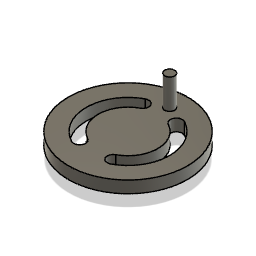
Quick Return Mechanism_ (Autodesk Fusion 360 design; units mm, degrees)
Autodesk Fusion 360 part; units mm, degrees
sketch "Sketch1" plane through (0, 0, 0) normal (0, 1, 0) x (1, 0, 0) in component "Fixed"
  arc A0 (32.0259, -54.4608) -> (60, 0) centre (-7, 0) ccw
  arc A1 (32.0259, -54.4608) -> (3, -110.75) centre (72.5197, -110.97) ccw
  line L0 (3, -110.75) -> (0, -110.75)
  line L1 (0, -110.75) -> (0, 0) construction
  circle A2 centre (30, -20) radius 15
  line L2 (0, -50.75) -> (25, -50.75)
  arc A3 (25, -50.75) -> (25, -40.75) centre (25, -45.75) ccw
  line L3 (25, -40.75) -> (15, -40.75)
  arc A4 (10, -35.75) -> (15, -40.75) centre (15, -35.75) ccw
  line L4 (10, -35.75) -> (10, -15.75)
  arc A5 (10, -15.75) -> (0, -5.75) centre (0, -15.75) ccw
  line L5 (30, -45.75) -> (30, -20) construction
  line L6 (60, 0) -> (0, 0)
  line L7 (0, 0) -> (0, 11.5) construction
  line L8 (0, 11.5) -> (60, 11.5)
  line L9 (60, 11.5) -> (60, 0)
  line L10 (60, 9) -> (0, 9)
  circle A6 centre (0, -65.75) radius 6
  circle A7 centre (0, -100.75) radius 2.05
  line L11 (-2.5, -78.25) -> (-2.5, -93.25)
  arc A8 (-2.5, -93.25) -> (2.5, -93.25) centre (0, -93.25) ccw
  line L12 (2.5, -93.25) -> (2.5, -78.25)
  arc A9 (2.5, -78.25) -> (-2.5, -78.25) centre (0, -78.25) ccw
  line L13 (0, -78.25) -> (0, -93.25) construction
  line L14 (-3, -110.75) -> (0, -110.75)
  arc A10 (-3, -110.75) -> (-32.0259, -54.4608) centre (-72.5197, -110.97) ccw
  arc A11 (-60, 0) -> (-32.0259, -54.4608) centre (7, 0) ccw
  arc A12 (-25, -40.75) -> (-25, -50.75) centre (-25, -45.75) ccw
  line L15 (-25, -40.75) -> (-15, -40.75)
  arc A13 (-15, -40.75) -> (-10, -35.75) centre (-15, -35.75) ccw
  line L16 (-10, -35.75) -> (-10, -15.75)
  arc A14 (0, -5.75) -> (-10, -15.75) centre (0, -15.75) ccw
  line L17 (0, -50.75) -> (-25, -50.75)
  circle A15 centre (-30, -20) radius 15
  line L18 (-60, 0) -> (0, 0)
  line L19 (-60, 9) -> (0, 9)
  line L20 (0, 11.5) -> (-60, 11.5)
  line L21 (-60, 11.5) -> (-60, 0)
  point P0 (0, -85.75)
  dimension "d1" = 7
  dimension "d2" = 67
  dimension "d3" = 69.52
  dimension "d4" = 110.75
  dimension "d5" = 3
  dimension "d6" = 30
  dimension "d7" = 20
  dimension "d8" = 5
  dimension "d9" = 10
  dimension "d10" = 5
  dimension "d11" = 10
  dimension "d12" = 25
  dimension "d13" = 15.75
  dimension "d14" = 90.75
  dimension "d15" = 11.5
  dimension "d16" = 9
  dimension "d17" = 12
  dimension "d18" = 4.1
  dimension "d19" = 2.5
  dimension "d20" = 10
  dimension "d21" = 15
  dimension "d22" = 45
  dimension "d23" = 25
  constraint tangent A0 A1
  constraint horizontal L1.end A0.centre
  constraint horizontal L0
  constraint coincident L1.end L6.end
  constraint vertical L1
  constraint horizontal L1.end A0.end
  constraint coincident L1 L2.start
  constraint perpendicular L1 L2
  constraint tangent L2 A3
  constraint tangent A3 L3
  constraint parallel L2 L3
  constraint tangent L3 A4
  constraint tangent A4 L4
  constraint coincident L1 A5.end
  constraint tangent L4 A5
  constraint vertical L4
  constraint midpoint A3 L5.start
  constraint coincident A2.centre L5.end
  constraint vertical L5
  constraint horizontal L6
  constraint vertical L7
  constraint horizontal L8
  constraint vertical L9
  constraint coincident L1.end L7
  constraint coincident L9 L10.start
  constraint coincident L7 L10.end
  constraint perpendicular L7 L10
  constraint coincident L1 A6.centre
  constraint coincident L1 A7.centre
  constraint tangent L11 A8
  constraint tangent A8 L12
  constraint parallel L11 L12
  constraint tangent L12 A9
  constraint tangent L11 A9
  constraint coincident L1 A8.centre
  constraint parallel L1 L13
  constraint coincident L1 P0
  constraint midpoint L13 P0
  constraint symmetric A0.start L7 A10.end
  constraint symmetric A0.end L7 A11.start
  constraint symmetric A0 L7 A11
  constraint symmetric A1.end L7 L14.start
  constraint symmetric A1 L7 A10
  constraint symmetric L0.end L7 L1.start
  constraint symmetric A2 L7 A15
  constraint symmetric L2.start L7 L17.start
  constraint symmetric L2.end L7 A12.end
  constraint symmetric A3.end L7 A12.start
  constraint symmetric A3 L7 A12
  constraint symmetric L3.end L7 L15.end
  constraint symmetric A4.start L7 A13.end
  constraint symmetric A4 L7 A13
  constraint symmetric L4.end L7 L16.end
  constraint symmetric A5.end L7 A14.start
  constraint symmetric A5 L7 A14
  constraint symmetric L1.end L7 L6.end
  constraint symmetric L8.start L7 L20.start
  constraint symmetric L8.end L7 L20.end
  constraint symmetric L7 L10.start L19.start
  constraint symmetric L7 L10.end L19.end
  measures "d1" distance of L1.end A0.centre
  measures "d2" radius of A0
  measures "d3" radius of A1
  measures "d4" vertical distance of L1.end A1.end
  measures "d5" distance of A1.end L0.end
  measures "d6" diameter of A2
  measures "d7" distance of A4.start L4.end
  measures "d8" radius of A3
  measures "d9" distance of A3.end L3.end
  measures "d10" radius of A4
  measures "d11" radius of A5
  measures "d12" distance of L2.start L2.end
  measures "d13" distance of L1.end A5.centre
  measures "d14" vertical distance of A1.end A2.centre
  measures "d15" distance of A0.end L8.end
  measures "d16" distance of A0.end L10
  measures "d17" diameter of A6
  measures "d18" diameter of A7
  measures "d19" radius of A9
  measures "d20" vertical distance of A1.end A7.centre
  measures "d21" distance of A8.end L12.end
  measures "d22" vertical distance of A1.end A6.centre
  measures "d23" vertical distance of A1.end P0
extrude "Extrude1" add sketch "Sketch1" along normal blind 5 contours A0 A1 L0 L6 L14 A10 A11 L18 | L6 L9 L10 L18 L19 L21 | L8 L9 L10 L19 L20 L21 | A7 makes body 1 in component "Fixed"
extrude "Extrude2" cut sketch "Sketch1" against normal blind 2.5 from surface at 5 contours L6 L9 L10 L18 L19 L21 bodies 1 in component "Fixed"
extrude "Extrude3" add sketch "Sketch1" along normal blind 25 contours A7 bodies 1 in component "Fixed"
sketch "Sketch1 (2)" plane through (0, 0, 0) normal (0, 1, 0) x (1, 0, 0) in component "Crank"
  circle A0 centre (0, -65.75) radius 6
  circle A1 centre (0, -65.75) radius 5.65
  dimension "d31" = 11.3
  constraint concentric A0 A1
  measures "d31" diameter of A1
extrude "Extrude1'" add sketch "Sketch1 (2)" along normal blind 5 separate body contours A1 makes body 2 in component "Crank"
sketch "Sketch2" plane through (0, 5, 0) normal (0, 1, 0) x (-1, 0, 0) in component "Crank"
  circle A0 centre (0, 65.75) radius 5.65
  circle A1 centre (0, 65.75) radius 25
  arc A2 (-8.2158, 81.2016) -> (-8.2158, 50.2984) centre (0, 65.75) ccw
  arc A3 (-5.8684, 76.7868) -> (-8.2158, 81.2016) centre (-7.0421, 78.9942) ccw
  arc A4 (-5.8684, 76.7868) -> (-5.8684, 54.7132) centre (0, 65.75) ccw
  arc A5 (-8.2158, 50.2984) -> (-5.8684, 54.7132) centre (-7.0421, 52.5058) ccw
  arc A6 (-7.0421, 78.9942) -> (-7.0421, 52.5058) centre (0, 65.75) ccw construction
  line L0 (-7.0421, 52.5058) -> (0, 65.75) construction
  line L1 (0, 65.75) -> (-7.0421, 78.9942) construction
  line L2 (0, 65.75) -> (0, 40.75) construction
  arc A7 (5.8684, 54.7132) -> (8.2158, 50.2984) centre (7.0421, 52.5058) ccw
  arc A8 (8.2158, 50.2984) -> (8.2158, 81.2016) centre (0, 65.75) ccw
  arc A9 (8.2158, 81.2016) -> (5.8684, 76.7868) centre (7.0421, 78.9942) ccw
  arc A10 (5.8684, 54.7132) -> (5.8684, 76.7868) centre (0, 65.75) ccw
  line L3 (7.0421, 52.5058) -> (0, 65.75) construction
  circle A11 centre (0, 48.25) radius 2.1
  dimension "d34" = 50
  dimension "d35" = 124
  dimension "d36" = 17.5
  dimension "d37" = 12.5
  dimension "d38" = 56
  dimension "d39" = 4.2
  dimension "d40" = 17.5
  constraint concentric A0 A1
  constraint tangent A2 A3
  constraint tangent A3 A4
  constraint tangent A4 A5
  constraint tangent A2 A5
  constraint coincident A0.centre A1.centre
  constraint coincident A5.centre A6.end
  constraint coincident A3.centre A6.start
  constraint coincident A1 L2.end
  constraint vertical L2
  constraint symmetric A2.end L2 A7.end
  constraint symmetric A2.start L2 A8.end
  constraint symmetric A3.start L2 A9.end
  constraint symmetric A4.end L2 A7.start
  constraint symmetric A2 L2 A8
  constraint symmetric A3 L2 A9
  constraint symmetric A4 L2 A10
  constraint symmetric A5 L2 A7
  constraint symmetric A5.centre L2 A7.centre
  constraint symmetric A0.centre L2 A1.centre
  constraint coincident L2 A11.centre
  measures "d34" diameter of A1
  measures "d35" angle of L0 L1
  measures "d36" radius of A2
  measures "d37" radius of A4
  measures "d38" angle of L0 L3
  measures "d39" diameter of A11
  measures "d40" distance of A0.centre A11.centre
extrude "Extrude2'" add sketch "Sketch2" along normal blind 5 separate body contours A0 | A1 | A11 makes body 3 in component "Crank"
extrude "Extrude3'" add sketch "Sketch2" along normal blind 17.5 contours A11 bodies 3 in component "Crank"
sketch "Sketch1 (3)" plane through (0, 10, 0) normal (0, 1, 0) x (-1, 0, 0) in component "FrontLever"
  circle A0 centre (0, 48.25) radius 2.1
  arc A1 (-5.8684, 76.7868) -> (-8.2158, 81.2016) centre (-7.0421, 78.9942) ccw
  arc A2 (-5.8684, 76.7868) -> (-5.8684, 54.7132) centre (0, 65.75) ccw
  arc A3 (-8.2158, 50.2984) -> (-5.8684, 54.7132) centre (-7.0421, 52.5058) ccw
  arc A4 (-8.2158, 81.2016) -> (-8.2158, 50.2984) centre (0, 65.75) ccw
  arc A5 (8.2158, 50.2984) -> (8.2158, 81.2016) centre (0, 65.75) ccw
  arc A6 (5.8684, 54.7132) -> (8.2158, 50.2984) centre (7.0421, 52.5058) ccw
  arc A7 (5.8684, 54.7132) -> (5.8684, 76.7868) centre (0, 65.75) ccw
  arc A8 (8.2158, 81.2016) -> (5.8684, 76.7868) centre (7.0421, 78.9942) ccw
  circle A9 centre (0, 65.75) radius 25
  circle A10 centre (0, 100.75) radius 2.05
  circle A11 centre (0, 100.75) radius 2.5
  line L0 (6.5, 20.75) -> (-6.5, 20.75)
  line L1 (-6.5, 20.75) -> (-6.5, 100.75)
  line L2 (6.5, 100.75) -> (6.5, 20.75)
  arc A12 (6.5, 100.75) -> (-6.5, 100.75) centre (0, 100.75) ccw
  arc A13 (-2.5, 94.75) -> (2.5, 94.75) centre (0, 100.75) ccw
  line L3 (2.5, 94.75) -> (-2.5, 94.75)
  line L4 (-2.5, 94.75) -> (-2.5, 33.25)
  line L5 (-2.5, 33.25) -> (2.5, 33.25)
  line L6 (2.5, 33.25) -> (2.5, 94.75)
  circle A14 centre (0, 26.25) radius 2.25
  dimension "d45" = 5
  dimension "d47" = 13
  dimension "d48" = 6.5
  dimension "d49" = 5
  dimension "d50" = 12.5
  dimension "d51" = 61.5
  dimension "d52" = 4.5
  dimension "d53" = 5.5
  constraint concentric A10 A11
  constraint horizontal L0
  constraint vertical L1
  constraint vertical L2
  constraint tangent L2 A12
  constraint coincident A10.centre A11.centre
  constraint horizontal L3
  constraint vertical L4
  constraint horizontal L5
  constraint vertical L6
  constraint coincident A13.end L3.start
  constraint coincident A13.start L3.end
  constraint equal A12 A13
  constraint vertical A10.centre A14.centre
  measures "d45" diameter of A11
  measures "d47" distance of L1 L2
  measures "d48" radius of A12
  measures "d49" distance of L4.end L5.end
  measures "d50" distance of L0 L5
  measures "d51" distance of A13.start L4.end
  measures "d52" diameter of A14
  measures "d53" distance of L0 A14.centre
extrude "Extrude1''" add sketch "Sketch1 (3)" along normal blind 5 separate body contours A1 A2 L1 | A1 A2 A3 A9 L1 L4 | A9 L1 L2 A12 L3 L4 L6 | A2 A3 L1 | A9 L0 L1 L2 L4 L5 L6 | A6 A7 A8 A9 L2 L6 | A13 L3 | A7 A8 L2 | A6 A7 L2 makes body 4 in component "FrontLever"
extrude "Extrude2''" add sketch "Sketch1 (3)" along normal blind 20 contours A14 bodies 4 in component "FrontLever"
sketch "Sketch1 (4)" plane through (0, 2.5, 0) normal (0, 1, 0) x (-1, 0, 0) in component "Slider"
  line L0 (60, -9) -> (60, 0)
  line L1 (60, 0) -> (-60, 0)
  line L2 (-60, 0) -> (-60, -9)
  line L3 (-60, -9) -> (60, -9)
  line L4 (20, -0.5) -> (-100, -0.5)
  line L5 (-100, -0.5) -> (-100, -8.5)
  line L6 (-100, -8.5) -> (20, -8.5)
  line L7 (20, -8.5) -> (20, -0.5)
  circle A0 centre (10, -4.5) radius 2.1
  circle A1 centre (10, -4.5) radius 3
  line L8 (10, -4.5) -> (20, -4.5) construction
  dimension "d86" = 120
  dimension "d87" = 8
  dimension "d88" = 0.5
  dimension "d101" = 4.2
  dimension "d102" = 40
  dimension "d103" = 10
  dimension "d104" = 6
  constraint horizontal L4
  constraint vertical L5
  constraint horizontal L6
  constraint vertical L7
  constraint coincident L4.start L7.end
  constraint concentric A0 A1
  constraint coincident A0.centre A1.centre
  constraint midpoint L7 L8.end
  constraint horizontal L8
  measures "d86" distance of L5.end L6.end
  measures "d87" distance of L4.start L6.end
  measures "d88" vertical distance of L1.end L4.end
  measures "d101" diameter of A0
  measures "d102" horizontal distance of L0.end L4.start
  measures "d103" distance of L7 A0.centre
  measures "d104" diameter of A1
extrude "Extrude1'''" add sketch "Sketch1 (4)" along normal blind 2.5 separate body contours L2 L4 L5 L6 | L2 L4 L6 L7 | A0 | A1 makes body 5 in component "Slider"
extrude "Extrude2'''" add sketch "Sketch1 (4)" along normal blind 12.5 contours A1 bodies 5 in component "Slider"
extrude "Extrude3''" add sketch "Sketch1 (4)" along normal blind 17.5 contours A0 bodies 5 in component "Slider"
sketch "Sketch1 (5)" plane through (0, 15, 0) normal (0, 1, 0) x (-1, 0, 0) in component "ConRod"
  circle A0 centre (10, -4.5) radius 2.1
  circle A1 centre (10, -4.5) radius 3
  line L0 (14, -4.5) -> (14, 54.07)
  arc A2 (14, 54.07) -> (6, 54.07) centre (10, 54.07) ccw
  line L1 (6, 54.07) -> (6, -4.5)
  arc A3 (6, -4.5) -> (14, -4.5) centre (10, -4.5) ccw
  line L2 (10, -4.5) -> (10, 54.07) construction
  circle A4 centre (10, -4.5) radius 2.5
  circle A5 centre (10, 54.07) radius 2.5
  dimension "d112" = 58.57
  dimension "d113" = 5
  dimension "d114" = 4
  dimension "d115" = 5
  constraint tangent L0 A2
  constraint tangent A2 L1
  constraint parallel L0 L1
  constraint tangent L1 A3
  constraint tangent L0 A3
  constraint coincident A0.centre A1.centre
  constraint concentric A3 A4
  constraint concentric A2 A5
  constraint vertical L2
  measures "d112" distance of A0.centre A2.centre
  measures "d113" diameter of A4
  measures "d114" radius of A3
  measures "d115" diameter of A5
extrude "Extrude1''''" add sketch "Sketch1 (5)" along normal blind 5 separate body contours L0 A2 L1 A3 makes body 6 in component "ConRod"
combine "Combine1" operation add target body 2 tool bodies 3 in component "Crank"
component "Fixed" placed x (1, 0, 0) y (0, 1, 0) z (0, 0, 1) at (0, 0, 0)
component "Crank" placed x (1, 0, 0) y (0, 1, 0) z (0, 0, 1) at (0, 0, 0)
component "FrontLever" placed x (1, 0, 0) y (0, 1, 0) z (0, 0, 1) at (0, 0, 0)
component "Slider" placed x (1, 0, 0) y (0, 1, 0) z (0, 0, 1) at (-39.8486, 0, 0)
component "ConRod" placed x (0.525013, 0, -0.851094) y (0, 1, 0) z (0.851094, 0, 0.525013) at (-40.7685, 0, -10.6484)
equation "d4 = 122.25 mm - 11.5 mm"
equation "d43 = 12.5 mm + 5 mm"
equation "d47 = ( 6.5 * 2 ) * 1 mm"
equation "d56 = 15 mm + 5 mm"
equation "d92 = ( 5 * -1 ) * 1 mm"
equation "d109 = 15 mm + 2.5 mm"
